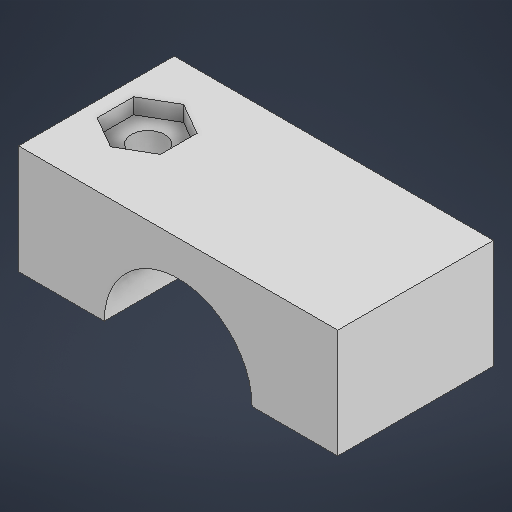
# Autodesk Inventor part: dg_clampv2
Saved by Autodesk Inventor 2026.1 (Build 301233020, 233B)
## iProperties
Created: 2026-03-08
Part Number: dg_clampv2
Material: Generic
Document SubType Name: Modeling
Designer: Dylan
Density: 1 g/cm^3
Appearance: Default
Author: Dylan
Autodesk Inventor part; units mm, degrees
ref_plane "YZ Plane" through (0, 0, 0) normal (1, 0, 0) x (0, 1, 0)
ref_plane "XZ Plane" through (0, 0, 0) normal (0, 1, 0) x (-1, 0, 0)
ref_plane "XY Plane" through (0, 0, 0) normal (0, 0, 1) x (1, 0, 0)
sketch "Sketch1" plane through (0, 0, 0) normal (0, 1, 0) x (-1, 0, 0)
  line L0 (0, 0) -> (-20.51, 0)
  line L1 (-20.51, 0) -> (-20.51, -10)
  line L2 (-20.51, -10) -> (0, -10)
  line L3 (0, -10) -> (0, 0)
  dimension "d0" = 20.51
  dimension "d1" = 10
  constraints: 8 end point, 2 parallel, 1 horizontal, 1 perpendicular
  measures "d0" distance of L2.end L1.end
  measures "d1" distance of L1.end L0.end
extrude "Extrusion1" add sketch "Sketch1" along normal blind 7
sketch "Sketch2" plane through (0, 0, 0) normal (0, 0, 1) x (1, 0, 0)
  line L0 (20.51, 0) -> (0, 0) projected
  circle A0 centre (10.255, 0) radius 4.75
  dimension "d4" = 9.5
  constraints: 1 centre point, 1 midpoint
  measures "d4" diameter of A0
extrude "Extrusion2" cut sketch "Sketch2" against normal through all
sketch "Sketch3" plane through (0, 7, 0) normal (0, 1, 0) x (1, 0, 0)
  line L0 (3, 7.6072) -> (5.0352, 6.4322)
  line L1 (5.0352, 6.4322) -> (5.0352, 4.0822)
  line L2 (5.0352, 4.0822) -> (3, 2.9072)
  line L3 (3, 2.9072) -> (0.9648, 4.0822)
  line L4 (0.9648, 4.0822) -> (0.9648, 6.4322)
  line L5 (0.9648, 6.4322) -> (3, 7.6072)
  point P0 (0, 0)
  point P1 (3, 5.2572)
  constraints: 12 end point, 13 other
extrude "Extrusion3" cut sketch "Sketch3" against normal blind 1
sketch "Sketch4" plane through (0, 6, 0) normal (0, 1, 0) x (1, 0, 0)
  circle A0 centre (3.0647, 5.2572) radius 1.075
  point P0 (0, 0)
  dimension "d10" = 2.15
  constraints: 1 centre point
  measures "d10" diameter of A0
extrude "Extrusion4" cut sketch "Sketch4" against normal through all
body "Solid1"
